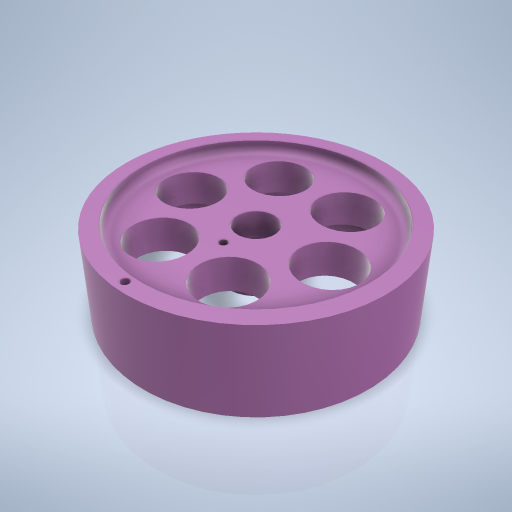
# Autodesk Inventor part: schwingrad
Saved by Autodesk Inventor 2024.2 (Build 282272000, 272)
## iProperties
Created: 2024-04-15
Part Number: schwingrad
Material: Polypropylen
Document SubType Name: Modeling
Designer: Fabri
Density: 0.899 g/cm^3
Appearance: Glatt - Violett
Author: Fabri
Autodesk Inventor part; units mm, degrees
ref_plane "YZ Plane" through (0, 0, 0) normal (1, 0, 0) x (0, 1, 0)
ref_plane "XZ Plane" through (0, 0, 0) normal (0, 1, 0) x (-1, 0, 0)
ref_plane "XY Plane" through (0, 0, 0) normal (0, 0, 1) x (1, 0, 0)
sketch "Skizze1" plane through (0, 0, 0) normal (0, 0, 1) x (1, 0, 0)
  circle A0 centre (0, 0) radius 34
  dimension "d0" = 68
  constraints: 1 centre point, 1 coincident
  measures "d0" diameter of A0
extrude "Extrusion1" add sketch "Skizze1" along normal mid plane 21
sketch "Skizze2" plane through (0, 0, 10.5) normal (0, 0, 1) x (1, 0, 0)
  circle A0 centre (0, 0) radius 30
  dimension "d3" = 60
  constraints: 1 centre point, 1 coincident
  measures "d3" diameter of A0
extrude "Extrusion2" cut sketch "Skizze2" against normal blind 3
fillet "Rundung1" radius 2 1 edges at (-30, 0, 7.5)
sketch "Skizze3" plane through (0, 0, -10.5) normal (0, 0, -1) x (-1, 0, 0)
  circle A0 centre (0, 0) radius 30
  dimension "d7" = 60
  constraints: 1 centre point, 1 coincident
  measures "d7" diameter of A0
extrude "Extrusion3" cut sketch "Skizze3" against normal blind 10
fillet "Rundung2" radius 2 1 edges at (30, 0, -0.5)
sketch "Skizze4" plane through (0, 0, -0.5) normal (0, 0, -1) x (-1, 0, 0)
  circle A0 centre (0, 0) radius 8
  dimension "d11" = 16
  constraints: 1 centre point, 1 coincident
  measures "d11" diameter of A0
extrude "Extrusion4" add sketch "Skizze4" along normal blind 3.5
sketch "Skizze5" plane through (0, 0, -4) normal (0, 0, -1) x (-1, 0, 0)
  circle A0 centre (0, 0) radius 8 projected
  constraints: 1 coincident
hole "Bohrung1" at (0, 0, -4) direction (0, 0, 1) diameter 10 depth 11.5
sketch "Skizze6" plane through (0, 0, -0.5) normal (0, 0, -1) x (-1, 0, 0)
  circle A0 centre (0, 0) radius 8 projected
  line L0 (0, 0) -> (0, 46.0089) construction
  circle A1 centre (0, 0) radius 5 projected
  line L1 (0, 0) -> (-23.7907, 41.2067) construction
  circle A2 centre (0, 0) radius 19 construction
  point P0 (-9.5, 16.4545)
  dimension "d22" = 38
  dimension "d21" = 30
  constraints: 4 end point, 1 coincident, 1 point on line, 1 vertical, 3 other
  measures "d21" angle of L0 L1
hole "Bohrung2" at (9.5, 16.4545, -0.5) direction (0, 0, 1) diameter 15 depth 8
pattern_circular "Runde Anordnung1" count 6 over 360 about axis through (0, 0, -10.5) along (0, 0, 1) of "Bohrung2"
sketch "Skizze7" plane through (0, 0, -10.5) normal (0, 0, -1) x (-1, 0, 0)
  point P0 (0, 0)
  point P1 (0, -31.75)
  dimension "d40" = 31.75
  constraints: 1 vertical alignment
  measures "d40" distance of point (0, -31.75) point (0, 0)
hole "Bohrung3" at (0, -31.75, -10.5) direction (0, 0, 1) diameter 2 end through all
sketch "Skizze8" plane through (0, 0, 7.5) normal (0, 0, 1) x (1, 0, 0)
  point P0 (0, 0)
  point P1 (0, -8.75)
  dimension "d48" = 8.75
  constraints: 1 vertical alignment
  measures "d48" distance of point (0, -8.75) point (0, 0)
hole "Bohrung4" at (0, -8.75, 7.5) direction (0, 0, -1) diameter 2 end through all
